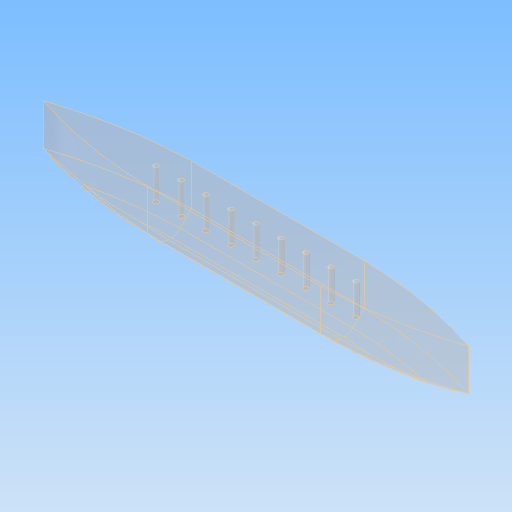
# Autodesk Inventor part: Außenrumpf_schnittig
Saved by Autodesk Inventor 2024.4 (Build 284460000, 460)
## iProperties
Created: 2026-01-18
Part Number: Außenrumpf_schnittig
Material: Polycarbonat, rauchfarben
Document SubType Name: Modeling
Designer: windows-desktop
Mass: 449392 g
Surface Area: 47086.2 cm^2
Volume: 374493 cm^3
Density: 1.2 g/cm^3
Appearance: Polycarbonat - Rauch
Masse[kg]: 449,4 kg
Autodesk Inventor part; units mm, degrees
ref_plane "YZ Plane" through (0, 0, 0) normal (1, 0, 0) x (0, 1, 0)
ref_plane "XZ Plane" through (0, 0, 0) normal (0, 1, 0) x (-1, 0, 0)
ref_plane "XY Plane" through (0, 0, 0) normal (0, 0, 1) x (1, 0, 0)
sketch "Skizze1" plane through (0, 0, 0) normal (0, 0, 1) x (1, 0, 0)
  line L0 (-1700, 175) -> (1700, 175)
  line L1 (1700, 175) -> (1700, -175)
  line L2 (1700, -175) -> (-1700, -175)
  line L3 (-1700, -175) -> (-1700, 175)
  line L4 (-2389.1597, 0) -> (2389.1597, 0) construction
  line L5 (0, -4575.1878) -> (0, 4575.1878) construction
  arc A0 (690.7597, -175) -> (1700, 0) centre (613.5452, 3267.9913) ccw
  arc A1 (-1700, 0) -> (-690.7597, -175) centre (-613.5452, 3267.9913) ccw
  arc A2 (1700, 0) -> (690.7597, 175) centre (613.5452, -3267.9913) ccw
  arc A3 (-690.7597, 175) -> (-1700, 0) centre (-613.5452, -3267.9913) ccw
  point P0 (0, 0)
  point P1 (-723.4779, 175)
  point P2 (-137.1412, -175)
  point P3 (-375.217, 175)
  point P4 (-690.7597, 175)
  point P5 (-690.7597, -175)
  point P6 (690.7597, 175)
  dimension "d0" = 3400
  dimension "d1" = 350
  constraints: 8 end point, 8 point on circle, 6 point on line, 6 symmetric about line, 4 centre point, 2 midpoint, 2 parallel, 1 horizontal, 1 perpendicular, 5 other
  measures "d0" distance of L1.end L2.end
  measures "d1" distance of L0.end L1.end
extrude "Extrusion1" add sketch "Skizze1" along normal blind 450 contours L0 A2 A0 L2 A1 A3
sketch "Skizze2" plane through (0, 0, 450) normal (0, 0, 1) x (1, 0, 0)
  line L0 (875.2225, 67.5814) -> (-875.2225, 67.5814) construction
  line L1 (0, 0) -> (-800, 0)
  circle A0 centre (800, 0) radius 20
  line L2 (800, 0) -> (-800, 0)
  line L3 (823.8178, -79.3063) -> (-823.8178, -79.3063) construction
  line L4 (800, 0) -> (2400, 0) construction
  circle A1 centre (600, 0) radius 20
  circle A2 centre (400, 0) radius 20
  circle A3 centre (200, 0) radius 20
  circle A4 centre (0, 0) radius 20
  circle A5 centre (-200, 0) radius 20
  circle A6 centre (-400, 0) radius 20
  circle A7 centre (-600, 0) radius 20
  circle A8 centre (-800, 0) radius 20
  point P0 (850.2799, 32.5814)
  point P1 (-850.2799, 32.5814)
  point P2 (851.0913, -44.3063)
  point P3 (-851.0913, -44.3063)
  point P4 (1100, 67.5814)
  point P5 (-1100, 67.5814)
  point P6 (1100, -79.3063)
  point P7 (-1100, -79.3063)
  point P8 (-875.2225, 67.5814)
  point P9 (-823.8178, -79.3063)
  dimension "d19" = 40
  dimension "d21" = 1600
  dimension "d22" = 180
  dimension "d28" = 200
  constraints: 9 centre point, 6 end point, 4 horizontal, 1 collinear, 18 other
  measures "d19" diameter of A0
  measures "d21" distance of L2.start L1.end
  measures "d22" angle of L2 L4
  measures "d28" distance of L2.start A1.centre
extrude "Extrusion2" cut sketch "Skizze2" against normal blind 250
chamfer "Fasen8" distance 120 angle 45 6 edges at (1201.9225, 125.2318, 0) (1201.9225, -125.2318, 0) (0, 175, 0) (0, -175, 0) (-1201.9225, 125.2318, 0) (-1201.9225, -125.2318, 0)
fillet "Rundung7" radius 100 6 edges at (956.0012, 38.1771, 0) (956.0012, -38.1771, 0) (0, 55, 0) (0, -55, 0) (-956.0012, 38.1771, 0) (-956.0012, -38.1771, 0)
